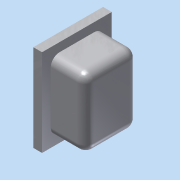
# Autodesk Inventor part: Button
Saved by Autodesk Inventor 2015 (Build 190159000, 159)
## iProperties
Created: 2015-11-12
Part Number: Button
Material: ABS Plastic
Document SubType Name: Modeling
Designer: Raphael
Density: 1.06 g/cm^3
Appearance: Smooth - White
Author: Raphael
Autodesk Inventor part; units mm, degrees
ref_plane "YZ Plane" through (0, 0, 0) normal (1, 0, 0) x (0, 1, 0)
ref_plane "XZ Plane" through (0, 0, 0) normal (0, 1, 0) x (-1, 0, 0)
ref_plane "XY Plane" through (0, 0, 0) normal (0, 0, 1) x (1, 0, 0)
sketch "Sketch1" plane through (0, 0, 0) normal (1, 0, 0) x (0, 1, 0)
  line L0 (0, 0) -> (12.7, 0)
  line L1 (12.7, 0) -> (12.7, -9.525)
  line L2 (12.7, -9.525) -> (0, -9.525)
  line L3 (0, -9.525) -> (0, 0)
  dimension "d0" = 12.7
  dimension "d1" = 9.525
  constraints: 8 end point, 2 parallel, 1 horizontal, 1 perpendicular
  measures "d0" distance of L1.end L2.end
  measures "d1" distance of L0.end L1.end
extrude "Extrusion1" add sketch "Sketch1" along normal mid plane 6.35
sketch "Sketch2" plane through (-3.175, 0, 0) normal (-1, 0, 0) x (0, 0, 1)
  line L0 (0, 0) -> (0, 12.7) projected
  line L1 (0, 12.7) -> (-9.525, 12.7) projected
  line L2 (-9.525, 12.7) -> (-9.525, 0) projected
  line L3 (-9.525, 0) -> (0, 0) projected
  line L4 (1.5875, 14.2875) -> (1.5875, -1.5875)
  line L5 (1.5875, -1.5875) -> (-11.1125, -1.5875)
  line L6 (-11.1125, -1.5875) -> (-11.1125, 14.2875)
  line L7 (-11.1125, 14.2875) -> (1.5875, 14.2875)
  dimension "d4" = 1.5875
  constraints: 8 end point, 3 other
  measures "d4" distance between parallel lines of L0 L4
extrude "Extrusion2" add sketch "Sketch2" along normal blind 1.5875 contours L3 L2 L1 L0 | L4 L5 L6 L7
fillet "Fillet1" radius 1.5875 8 edges at (0, 12.7, 0) (3.175, 12.7, -4.7625) (0, 12.7, -9.525) (3.175, 6.35, -9.525) (0, 0, -9.525) (3.175, 0, -4.7625) (0, 0, 0) (3.175, 6.35, 0)
body "Solid1"
